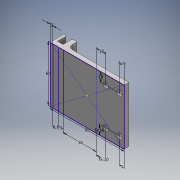
# Autodesk Inventor part: stabilisateur
Saved by Autodesk Inventor 2016 (Build 200138000, 138)
## iProperties
Created: 2018-04-26
Part Number: stabilisateur
Material: Generic
Document SubType Name: Modeling
Designer: mbouhier
Density: 1 g/cm^3
Appearance: Default
Author: mbouhier
Autodesk Inventor part; units mm, degrees
ref_plane "YZ Plane" through (0, 0, 0) normal (1, 0, 0) x (0, 1, 0)
ref_plane "XZ Plane" through (0, 0, 0) normal (0, 1, 0) x (-1, 0, 0)
ref_plane "XY Plane" through (0, 0, 0) normal (0, 0, 1) x (1, 0, 0)
sketch "Sketch1" plane through (0, 0, 0) normal (0, 1, 0) x (-1, 0, 0)
  line L0 (-40, 30) -> (40, 30)
  line L1 (40, 30) -> (40, -30)
  line L2 (40, -30) -> (-40, -30)
  line L3 (-40, -30) -> (-40, 30)
  line L4 (-40, 30) -> (40, -30) construction
  line L5 (40, 30) -> (-40, -30) construction
  line L6 (25.245, -30) -> (20.245, -30)
  line L7 (20.245, 30) -> (25.245, 30)
  line L8 (37, 30) -> (37, -30)
  line L9 (30.9, -30) -> (30.9, 30)
  line L10 (25.9, -30) -> (25.9, 30)
  line L11 (-10.1, -30) -> (-10.1, 30) construction
  point P0 (0, 0)
  point P1 (-35, 20)
  point P2 (-35, -20)
  point P3 (-20.1, 20)
  point P4 (-20.1, -20)
  dimension "d0" = 80
  dimension "d1" = 60
  dimension "d3" = 3
  dimension "d4" = 6.1
  dimension "d5" = 5
  dimension "d6" = 10
  dimension "d7" = 10
  dimension "d8" = 5
  dimension "d9" = 5
  dimension "d10" = 36
  dimension "d11" = 10
  dimension "d12" = 10
  constraints: 24 end point, 10 point on line, 5 perpendicular, 3 parallel, 2 horizontal, 2 midpoint
  measures "d0" distance of L1.end L2.end
  measures "d1" distance of L0.end L1.end
  measures "d3" distance between parallel lines of L8 L1
  measures "d4" distance between parallel lines of L9 L8
  measures "d5" distance between parallel lines of L10 L9
  measures "d6" distance from line of point (-35, 20) L0
  measures "d7" distance from line of L2 point (-35, -20)
  measures "d8" distance from line of point (-35, -20) L3
  measures "d9" distance from line of L3 point (-35, 20)
  measures "d10" distance between parallel lines of L11 L10
  measures "d11" distance from line of point (-20.1, 20) L11
  measures "d12" distance from line of point (-20.1, -20) L11
extrude "Extrusion1" add sketch "Sketch1" along normal blind 5
extrude "Extrusion2" add sketch "Sketch1" along normal blind 15 contours L0 L9 L2 L10 | L0 L1 L2 L8
chamfer "Chamfer1" distance 1 angle 45 2 edges at (-37, 15, 0) (-30.9, 15, 0)
fillet "Fillet1" radius 5 1 edges at (-25.9, 5, 0)
hole "Hole1" at (35, 0, 20) at (35, 0, -20) at (20.1, 0, 20) at (20.1, 0, -20) direction (0, 1, 0) diameter 3 end through all countersink diameter 6 countersink angle 90
equation "\"d7\" = d6"
equation "\"d9\" = d8"
equation "\"d12\" = d11"
body "Solid1"
